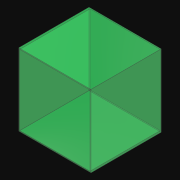
# Autodesk Inventor part: Sizing Tool
Saved by Autodesk Inventor 2021 (Build 250183000, 183)
## iProperties
Created: 2020-06-21
Part Number: Sizing Tool
Material: Generic
Document SubType Name: Modeling
Designer: yuany
Density: 1 g/cm^3
Appearance: Default
Author: yuany
Autodesk Inventor part; units mm, degrees
ref_plane "YZ Plane" through (0, 0, 0) normal (1, 0, 0) x (0, 1, 0)
ref_plane "XZ Plane" through (0, 0, 0) normal (0, 1, 0) x (-1, 0, 0)
ref_plane "XY Plane" through (0, 0, 0) normal (0, 0, 1) x (1, 0, 0)
sketch "Sketch1" plane through (0, 0, 0) normal (0, 0, 1) x (1, 0, 0)
  line L0 (0, 0) -> (469.9, 0)
  line L1 (469.9, 0) -> (469.9, 469.9)
  line L2 (469.9, 469.9) -> (0, 469.9)
  line L3 (0, 469.9) -> (0, 0)
  dimension "d0" = 469.9
  dimension "d1" = 469.9
  constraints: 8 end point, 2 parallel, 1 horizontal, 1 perpendicular
  measures "d0" distance of L2.end L1.end
  measures "d1" distance of L0.end L1.end
extrude "Extrusion1" add sketch "Sketch1" along normal blind 457.2
shell "Shell1" thickness 6.35 removed faces 2 at (156.6333, 313.2667, 0) at (156.6333, 313.2667, 457.2)
body "Solid1"
